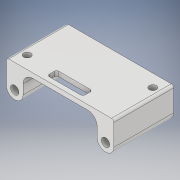
# Autodesk Inventor part: US Halterung hinten
Saved by Autodesk Inventor 2018 (Build 220112000, 112)
## iProperties
Created: 2019-03-05
Part Number: US Halterung hinten
Material: ABS-Kunststoff
Document SubType Name: Modeling
Designer: RedBots
Density: 0.732517 g/cm^3
Appearance: Glatt - weiß
Mass: 4 g
Surface Area: 43.527 cm^2
Volume: 5.46063 cm^3
Author: RedBots
Autodesk Inventor part; units mm, degrees
ref_plane "YZ Plane" through (0, 0, 0) normal (1, 0, 0) x (0, 1, 0)
ref_plane "XZ Plane" through (0, 0, 0) normal (0, 1, 0) x (-1, 0, 0)
ref_plane "XY Plane" through (0, 0, 0) normal (0, 0, 1) x (1, 0, 0)
sketch "Skizze1" plane through (0, 0, 0) normal (0, 0, 1) x (1, 0, 0)
  line L0 (0, 0) -> (45, 0)
  line L1 (45, 0) -> (45, 25)
  line L2 (45, 25) -> (0, 25)
  line L3 (0, 25) -> (0, 0)
  dimension "d5" = 45
  dimension "d6" = 25
  constraints: 8 end point, 2 parallel, 1 horizontal, 1 perpendicular
  measures "d5" distance of L1.end L2.end
  measures "d6" distance of L0.end L1.end
extrude "Extrusion1" add sketch "Skizze1" along normal blind 2
sketch "Skizze3" plane through (0, 25, 0) normal (0, 1, 0) x (1, 0, 0)
  circle A0 centre (3.5, 8) radius 1.75
  circle A1 centre (41.5, 8) radius 1.75
  line L0 (3.5, 8) -> (41.5, 8) construction
  line L1 (0, 0) -> (45, 0) construction
  line L2 (22.5, 0) -> (22.5, 8) construction
  line L3 (0, 0) -> (7, 0)
  line L4 (45, 0) -> (38, 0)
  line L5 (0, 0) -> (0, 8)
  line L6 (7, 8) -> (7, 0)
  line L7 (38, 8) -> (38, 0)
  line L8 (45, 0) -> (45, 8)
  arc A2 (7, 8) -> (0, 8) centre (3.5, 8) ccw
  arc A3 (45, 8) -> (38, 8) centre (41.5, 8) ccw
  dimension "d2" = 38
  dimension "d3" = 3.5
  dimension "d4" = 8
  constraints: 16 end point, 5 parallel, 4 centre point, 4 point on circle, 3 horizontal, 3 vertical, 2 coincident, 2 midpoint, 2 point on line, 1 equal radius
  measures "d2" distance of L0.start L0.end
  measures "d3" diameter of A0
  measures "d4" distance of L2.start L2.end
extrude "Extrusion2" add sketch "Skizze3" against normal up to surface (25 mm away)
sketch "Skizze4" plane through (0, 0, 2) normal (0, 0, 1) x (1, 0, 0)
  line L0 (3.45, 5.261) -> (41.55, 5.261) construction
  line L1 (41.55, 5.261) -> (41.55, 19.739) construction
  line L2 (41.55, 19.739) -> (3.45, 19.739) construction
  line L3 (3.45, 19.739) -> (3.45, 5.261) construction
  line L4 (45, 25) -> (0, 25) construction
  line L5 (22.5, 25) -> (22.5, 0) construction
  line L6 (0, 0) -> (45, 0) construction
  line L7 (0, 25) -> (0, 0) construction
  line L8 (0, 12.5) -> (45, 12.5) construction
  line L9 (45, 0) -> (45, 25) construction
  circle A0 centre (41.55, 19.739) radius 1.5
  circle A1 centre (3.45, 5.261) radius 1.5
  point P0 (22.5, 19.739)
  point P1 (41.55, 12.5)
  dimension "d12" = 38.1
  dimension "d13" = 14.478
  dimension "d14" = 3
  constraints: 12 end point, 6 midpoint, 2 centre point, 2 coincident, 2 parallel, 2 point on line, 1 equal radius, 1 horizontal, 1 perpendicular
  measures "d12" distance of L1.end L2.end
  measures "d13" distance between parallel lines of L0 L2
  measures "d14" diameter of A0
extrude "Extrusion3" cut sketch "Skizze4" against normal blind 8
sketch "Skizze5" plane through (0, 0, 2) normal (0, 0, 1) x (1, 0, 0)
  line L0 (44.09, 22.4949) -> (0.91, 22.4949) construction
  line L1 (0.91, 22.4949) -> (0.91, 2.5051) construction
  line L2 (0.91, 2.5051) -> (44.09, 2.5051) construction
  line L3 (44.09, 2.5051) -> (44.09, 22.4949) construction
  line L4 (45, 25) -> (0, 25) construction
  line L5 (22.5, 25) -> (22.5, 0) construction
  line L6 (0, 0) -> (45, 0) construction
  line L7 (45, 0) -> (45, 25) construction
  line L8 (45, 12.5) -> (0, 12.5) construction
  line L9 (0, 25) -> (0, 0) construction
  line L10 (15, 6.0051) -> (30, 6.0051)
  line L11 (30, 6.0051) -> (30, 2.0051)
  line L12 (30, 2.0051) -> (15, 2.0051)
  line L13 (15, 2.0051) -> (15, 6.0051)
  point P0 (0.91, 12.5)
  point P1 (22.5, 6.0051)
  dimension "d17" = 43.18
  dimension "d18" = 19.9898
  dimension "d19" = 15
  dimension "d20" = 4
  dimension "d27" = 0.5
  constraints: 20 end point, 6 midpoint, 4 parallel, 2 horizontal, 2 perpendicular, 2 point on line
  measures "d17" distance of L0.start L0.end
  measures "d18" distance of L0.end L1.end
  measures "d19" distance of L11.end L12.end
  measures "d20" distance of L10.end L11.end
  measures "d27" distance between parallel lines of L2 L12
extrude "Extrusion4" cut sketch "Skizze5" against normal up to next
fillet "Rundung1" radius 1 4 edges at (15, 6.0051, 1) (30, 6.0051, 1) (30, 2.0051, 1) (15, 2.0051, 1)
fillet "Rundung2" radius 4 2 edges at (7, 12.5, 0) (38, 12.5, 0)
fillet "Rundung3" radius 1 2 edges at (0, 12.5, 2) (45, 12.5, 2)
